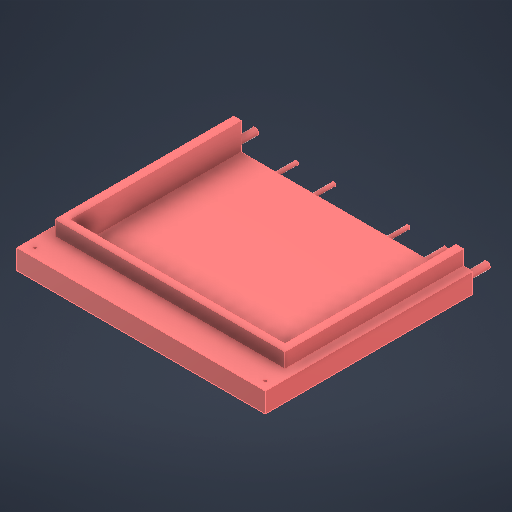
# Autodesk Inventor part: Enclosure 2 Bottom
Saved by Autodesk Inventor 2025.2 (Build 292293000, 293)
## iProperties
Created: 2025-02-10
Part Number: Enclosure 2 Bottom
Material: ABS Plastic
Document SubType Name: Modeling
Designer: elier
Density: 1.06 g/cm^3
Appearance: Smooth - Red
Author: elier
Autodesk Inventor part; units mm, degrees
ref_plane "YZ Plane" through (0, 0, 0) normal (1, 0, 0) x (0, 1, 0)
ref_plane "XZ Plane" through (0, 0, 0) normal (0, 1, 0) x (-1, 0, 0)
sketch "Sketch1" plane through (0, 0, 0) normal (0, 1, 0) x (-1, 0, 0)
  line L0 (-83.5, 139.5) -> (83.5, 139.5)
  line L1 (83.5, 139.5) -> (83.5, -139.5)
  line L2 (83.5, -139.5) -> (-83.5, -139.5)
  line L3 (-83.5, -139.5) -> (-83.5, 139.5)
  line L4 (-83.5, 139.5) -> (83.5, -139.5) construction
  line L5 (83.5, 139.5) -> (-83.5, -139.5) construction
  point P0 (0, 0)
  dimension "d0" = 167
  dimension "d1" = 279
  constraints: 12 end point, 2 midpoint, 2 parallel, 1 horizontal, 1 perpendicular
  measures "d0" distance of L1.end L2.end
  measures "d1" distance of L0.end L1.end
extrude "Extrusion1" add sketch "Sketch1" along normal blind 13.4
sketch "Sketch2" plane through (0, 13.4, 0) normal (0, 1, 0) x (1, 0, 0)
  line L0 (72.25, -115.05) -> (-72.25, -115.05)
  line L1 (-72.25, -115.05) -> (-72.25, 115.05)
  line L2 (-72.25, 115.05) -> (72.25, 115.05)
  line L3 (72.25, 115.05) -> (72.25, -115.05)
  line L4 (72.25, -115.05) -> (-72.25, 115.05) construction
  line L5 (-72.25, -115.05) -> (72.25, 115.05) construction
  point P0 (0, 0)
  dimension "d4" = 144.5
  dimension "d5" = 230.1
  constraints: 12 end point, 2 midpoint, 2 parallel, 1 horizontal, 1 perpendicular
  measures "d4" distance of L1.end L2.end
  measures "d5" distance of L0.end L1.end
extrude "Extrusion2" cut sketch "Sketch2" against normal blind 8.4
sketch "Sketch4" plane through (0, 13.4, 0) normal (0, 1, 0) x (1, 0, 0)
  circle A0 centre (-77.5, -133.5) radius 1.25
  line L0 (-83.5, 139.5) -> (-83.5, -139.5) projected
  line L1 (-83.5, -139.5) -> (83.5, -139.5) projected
  circle A1 centre (-77.5, 133.5) radius 1.25
  line L2 (83.5, 139.5) -> (-83.5, 139.5) projected
  circle A2 centre (77.5, 133.5) radius 1.25
  line L3 (83.5, -139.5) -> (83.5, 139.5) projected
  circle A3 centre (77.5, -133.5) radius 1.25
  point P0 (0, 0)
  dimension "d16" = 2.5
  dimension "d17" = 6
  dimension "d18" = 6
  dimension "d19" = 2.5
  dimension "d20" = 6
  dimension "d21" = 6
  dimension "d22" = 2.5
  dimension "d23" = 6
  dimension "d24" = 6
  dimension "d25" = 2.5
  dimension "d26" = 6
  dimension "d27" = 6
  constraints: 4 centre point
  measures "d16" diameter of A0
  measures "d17" distance from line of A0.centre L0
  measures "d18" distance from line of L1 A0.centre
  measures "d19" diameter of A1
  measures "d20" distance from line of L0 A1.centre
  measures "d21" distance from line of L2 A1.centre
  measures "d22" diameter of A2
  measures "d23" distance from line of L2 A2.centre
  measures "d24" distance from line of L3 A2.centre
  measures "d25" diameter of A3
  measures "d26" distance from line of L1 A3.centre
  measures "d27" distance from line of L3 A3.centre
extrude "Extrusion4" cut sketch "Sketch4" against normal through all contours A0 | A1 | A2 | A3
sketch "Sketch5" plane through (0, 13.4, 0) normal (0, 1, 0) x (1, 0, 0)
  line L0 (-72.25, -115.05) -> (-72.25, 115.05) projected
  line L1 (72.25, -115.05) -> (-72.25, -115.05) projected
  line L2 (-77.25, -120.05) -> (-72.25, -120.05)
  line L3 (-72.25, -120.05) -> (-72.25, 120.05)
  line L4 (-72.25, 120.05) -> (-77.25, 120.05)
  line L5 (-77.25, 120.05) -> (-77.25, -120.05)
  line L6 (72.25, 115.05) -> (72.25, -115.05) projected
  line L7 (77.25, -120.05) -> (72.25, -120.05)
  line L8 (72.25, -120.05) -> (72.25, 120.05)
  line L9 (72.25, 120.05) -> (77.25, 120.05)
  line L10 (77.25, 120.05) -> (77.25, -120.05)
  line L11 (-72.25, 115.05) -> (72.25, 115.05) projected
  line L12 (72.25, 120.05) -> (-72.25, 120.05)
  line L13 (-72.25, 120.05) -> (-72.25, 115.05)
  line L14 (-72.25, 115.05) -> (72.25, 115.05)
  line L15 (72.25, 115.05) -> (72.25, 120.05)
  line L16 (-72.25, -115.05) -> (72.25, -115.05)
  line L17 (72.25, -115.05) -> (72.25, -120.05)
  line L18 (72.25, -120.05) -> (-72.25, -120.05)
  line L19 (-72.25, -120.05) -> (-72.25, -115.05)
  point P0 (0, 0)
  dimension "d30" = 5
  dimension "d31" = 5
  dimension "d32" = 240.1
  dimension "d33" = 5
  dimension "d34" = 5
  dimension "d35" = 240.1
  constraints: 32 end point, 8 parallel, 4 horizontal, 4 perpendicular, 1 point on line
  measures "d30" distance from line of L0 L2.start
  measures "d31" distance from line of L1 L2.start
  measures "d32" distance of L3.end L2.end
  measures "d33" distance from line of L1 L7.start
  measures "d34" distance from line of L6 L7.start
  measures "d35" distance of L7.end L8.end
extrude "Extrusion5" add sketch "Sketch5" along normal blind 10 contours L3 L2 L5 L4 L0 | L1 L8 L18 L3 | L3 L12 L8 L11 | L6 L8 L9 L10 L7
sketch "Sketch7" plane through (0, 0, 0) normal (0, -1, 0) x (1, 0, 0)
  circle A0 centre (-77.5, -133.5) radius 1.25 projected
  circle A1 centre (-77.5, -133.5) radius 1.75
  circle A2 centre (-77.5, 133.5) radius 1.25 projected
  circle A3 centre (-77.5, 133.5) radius 1.75
  circle A4 centre (77.5, 133.5) radius 1.25 projected
  circle A5 centre (77.5, 133.5) radius 1.75
  circle A6 centre (77.5, -133.5) radius 1.25 projected
  circle A7 centre (77.5, -133.5) radius 1.75
  point P0 (0, 0)
  dimension "d42" = 3.5
  dimension "d43" = 3.5
  dimension "d44" = 3.5
  dimension "d45" = 3.5
  constraints: 4 centre point, 4 coincident
  measures "d42" diameter of A1
  measures "d43" diameter of A3
  measures "d44" diameter of A5
  measures "d45" diameter of A7
extrude "Extrusion6" cut sketch "Sketch7" against normal blind 11.4 contours A0 | A1 | A2 | A3 | A4 | A5 | A7
sketch "Sketch8" plane through (83.5, 0, 139.5) normal (1, 0, 0) x (0, 0, -1)
  line L0 (139.5, 0) -> (139.5, 13.4)
  line L1 (0, 13.4) -> (279, 13.4) projected
  constraints: 2 end point, 1 midpoint
sketch "Sketch9" plane through (0, 13.4, 0) normal (0, 1, 0) x (1, 0, 0)
  line L0 (83.5, -139.5) -> (83.5, 139.5) projected
  line L1 (83.5, 0) -> (77.25, 0)
  line L2 (77.25, 120.05) -> (77.25, -120.05) projected
  point P0 (0, 0)
  constraints: 2 end point, 2 midpoint
sketch "Sketch10" plane through (77.25, 13.4, 120.05) normal (1, 0, 0) x (0, 0, -1)
  line L0 (-19.45, 0) -> (259.55, 0) projected
  line L1 (120.05, 0) -> (120.05, 10)
  line L2 (0, 10) -> (240.1, 10) projected
  point P0 (120.05, -13.4)
  constraints: 2 end point, 2 midpoint
split_face "Split1"
split_face "Split2"
split_face "Split3"
ref_plane "Work Plane1" through (83.5, 0, -139.5) normal (1, 0, 0) x (0, 0, -1)
sketch "Sketch11" plane through (83.5, 0, -139.5) normal (1, 0, 0) x (0, 0, -1)
  line L0 (0, 0) -> (0, 13.4) projected
  line L1 (-139.5, 5) -> (-139.5, 23.4) projected
  line L2 (0, 0) -> (-139.5, 0)
  line L3 (-139.5, 0) -> (-139.5, 23.4)
  line L4 (-139.5, 23.4) -> (0, 23.4)
  line L5 (0, 23.4) -> (0, 0)
  point P0 (-139.5, 0)
  constraints: 8 end point, 2 parallel, 1 horizontal, 1 perpendicular
extrude "Extrusion7" cut sketch "Sketch11" against normal blind 167.1625
sketch "Sketch12" plane through (83.5, 0, 0) normal (0, 0, -1) x (-1, 0, 0)
  line L0 (0, 0) -> (0, 13.4) projected
  circle A0 centre (5.625, 6.7) radius 2.375
  line L1 (167, 0) -> (167, 13.4) projected
  circle A1 centre (161.375, 6.7) radius 2.375
  line L2 (11.25, 5) -> (155.75, 5) projected
  circle A2 centre (58.5, 2.5) radius 1.375
  circle A3 centre (33.5, 2.5) radius 1.375
  circle A4 centre (108.5, 2.5) radius 1.375
  circle A5 centre (133.5, 2.5) radius 1.375
  point P0 (83.5, 0)
  dimension "d51" = 4.75
  dimension "d53" = 4.75
  dimension "d55" = 2.75
  dimension "d57" = 2.75
  dimension "d59" = 2.75
  dimension "d61" = 2.75
  constraints: 6 centre point
  measures "d51" diameter of A0
  measures "d53" diameter of A1
  measures "d55" diameter of A2
  measures "d57" diameter of A3
  measures "d59" diameter of A4
  measures "d61" diameter of A5
extrude "Extrusion8" add sketch "Sketch12" along normal blind 15
body "Solid1"
